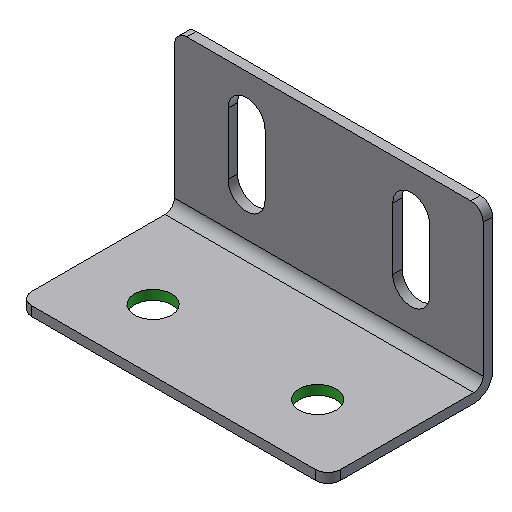
# Autodesk Inventor part: TL20240701-10130CV-003
Saved by Autodesk Inventor 2022.5 (Build 265521000, 521)
## iProperties
Category: JOINT LEG ASSY
Company: 현대 트랜시스(대유)
Created: 2023-04-20
Part Number: TL20240701-10130CV-003
Checked By: 김형민
Engr Approved By: 김시현
User Status: 2 x37
Material: SS400
Description: 0
Document SubType Name: Modeling
Mfg Approved By: 호상태
Designer: 김건휴
Density: 7.85 g/cm^3
Appearance: Painting-RAL7035
Project: SW PJT
Stock Number: 003
DETAIL: Coveryor Assembly
M/C TITLE: CJ 제일제당 협동로봇 포장시스탬 PILOT 장비
PARTS NAME: Bracket
SPECIFICATION: TA20221101-CV200000-015
DocNumber: 221118_Standard_v1
Folder: .\
VDS_Category: 엔지니어링
Detail Description: Processed products
Title: BRACKET
Subject: SW차종 시트조립라인
Author: 김건휴
Revision Number: B
Autodesk Inventor part; units mm, degrees
ref_plane "YZ Plane" through (0, 0, 0) normal (1, 0, 0) x (0, 1, 0)
ref_plane "XZ Plane" through (0, 0, 0) normal (0, 1, 0) x (-1, 0, 0)
ref_plane "XY Plane" through (0, 0, 0) normal (0, 0, 1) x (1, 0, 0)
sketch "스케치9" plane through (0, 0, 0) normal (1, 0, 0) x (0, 1, 0)
  line L0 (2.3, 0) -> (0, 0)
  line L1 (0, 0) -> (0, 40)
  line L2 (0, 40) -> (2.3, 40)
  line L3 (2.3, 40) -> (2.3, 0)
  line L4 (0, 0) -> (40, 0)
  line L5 (40, 0) -> (40, 2.3)
  line L6 (40, 2.3) -> (0, 2.3)
  line L7 (0, 2.3) -> (0, 0)
  point P0 (2.3, 2.3)
  dimension "d40" = 2.3
  dimension "d41" = 2.3
  dimension "d42" = 40
  dimension "d43" = 40
  constraints: 16 end point, 4 parallel, 2 horizontal, 2 perpendicular, 1 coincident
  measures "d40" distance of L4.end L5.end
  measures "d41" distance of L1.end L2.end
  measures "d42" distance of L0.end L1.end
  measures "d43" distance of L0.end L4.end
extrude "돌출4" add sketch "스케치9" along normal mid plane 75
sketch "스케치10" plane through (-37.5, 2.3, 40) normal (0, 1, 0) x (1, 0, 0)
  line L0 (0, 0) -> (0, 37.7) projected
  line L1 (0, 0) -> (75, 0) projected
  point P0 (37.5, 40)
  point P1 (17.5, 15)
  point P2 (57.5, 15)
  dimension "d46" = 40
  dimension "d47" = 17.5
  dimension "d48" = 15
  constraints: 1 horizontal alignment
  measures "d46" distance of point (57.5, 15) point (17.5, 15)
  measures "d47" distance from line of L0 point (17.5, 15)
  measures "d48" distance from line of L1 point (17.5, 15)
hole "구멍3" at (-20, 2.3, 25) at (20, 2.3, 25) direction (0, -1, 0) diameter 9 end through all clearance for "Socket Head Cap Screw ISO 4762" size "M8" standard "ISO"
sketch "스케치11" plane through (-37.5, 2.3, 2.3) normal (0, 0, 1) x (1, 0, 0)
  line L0 (0, 0) -> (0, 37.7) projected
  line L1 (75, 37.7) -> (0, 37.7) projected
  line L2 (57.5, 12.7) -> (57.5, 27.7) construction
  line L3 (62, 12.7) -> (62, 27.7)
  line L4 (53, 27.7) -> (53, 12.7)
  arc A0 (53, 12.7) -> (62, 12.7) centre (57.5, 12.7) ccw
  arc A1 (62, 27.7) -> (53, 27.7) centre (57.5, 27.7) ccw
  line L5 (17.5, 27.7) -> (17.5, 12.7) construction
  line L6 (13, 27.7) -> (13, 12.7)
  line L7 (22, 12.7) -> (22, 27.7)
  arc A2 (22, 27.7) -> (13, 27.7) centre (17.5, 27.7) ccw
  arc A3 (13, 12.7) -> (22, 12.7) centre (17.5, 12.7) ccw
  point P0 (37.5, -2.3)
  point P1 (17.5, 20.2)
  point P2 (57.5, 20.2)
  point P3 (0, -2.3)
  dimension "d56" = 17.5
  dimension "d57" = 40
  dimension "d69" = 7.5
  dimension "d70" = 9
  dimension "d71" = 7.5
  dimension "d72" = 9
  dimension "d73" = 22.5
  constraints: 16 end point, 8 point on circle, 8 tangent, 4 centre point, 3 parallel, 2 midpoint, 1 horizontal alignment, 1 vertical
  measures "d56" distance from line of L0 point (17.5, 20.2)
  measures "d57" distance of point (57.5, 20.2) point (17.5, 20.2)
  measures "d69" distance of point (57.5, 20.2) L2.end
  measures "d70" diameter of A1
  measures "d71" distance of point (17.5, 20.2) L5.end
  measures "d72" diameter of A3
  measures "d73" vertical distance of point (0, -2.3) point (17.5, 20.2)
fillet "모깎기2" radius 2.3 1 edges at (0, 2.3, 2.3)
fillet "모깎기3" radius 4.6 1 edges at (0, 0, 0)
fillet "모깎기4" radius 3 4 edges at (37.5, 40, 1.15) (-37.5, 40, 1.15) (37.5, 1.15, 40) (-37.5, 1.15, 40)
extrude "돌출5" cut sketch "스케치11" against normal blind 75
